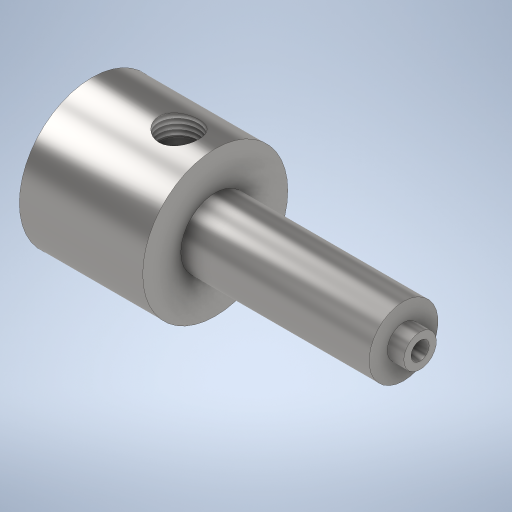
# Autodesk Inventor part: ASI Propane
Saved by Autodesk Inventor 2024 (Build 280153020, 153B)
## iProperties
Created: 2023-07-06
Part Number: ASI Propane
Material: Stainless Steel
Document SubType Name: Modeling
Designer: Victoria
Density: 8 g/cm^3
Appearance: Semi-Polished
Author: Victoria
Autodesk Inventor part; units mm, degrees
ref_plane "YZ Plane" through (0, 0, 0) normal (1, 0, 0) x (0, 1, 0)
ref_plane "XY Plane" through (0, 0, 0) normal (0, 0, 1) x (1, 0, 0)
sketch "Sketch1" plane through (0, 0, 0) normal (0, 0, 1) x (1, 0, 0)
  line L0 (0, 0) -> (0, 6.5)
  line L1 (0, 6.5) -> (54.81, 6.5)
  line L2 (67.887, 1.75) -> (54.81, 6.5)
  line L3 (71.47, 0) -> (71.47, 2.5)
  line L4 (71.47, 2.5) -> (67.887, 1.75)
  line L5 (0, 6.5) -> (0, 9.5)
  line L6 (0, 9.5) -> (60.7761, 9.5)
  line L7 (71.47, 0) -> (0, 0)
  line L8 (71.47, 2.5) -> (71.47, 4.5)
  line L9 (71.47, 4.5) -> (66.9088, 4.5)
  line L10 (66.9088, 4.5) -> (66.9088, 9.5)
  line L11 (66.9088, 9.5) -> (60.7761, 9.5)
  line L12 (66.9088, 9.5) -> (66.9088, 9.5)
  line L13 (66.9088, 9.5) -> (16.9088, 9.5)
  line L14 (16.9088, 9.5) -> (16.9088, 9.5)
  point P0 (71.47, 1.25)
  dimension "d0" = 6.5
  dimension "d1" = 54.81
  dimension "d5" = 2.5
  dimension "d6" = 3
  dimension "d7" = 0
  dimension "d8" = 50
  dimension "d44" = 1.75
  dimension "d45" = 3.583
  constraints: 30 end point, 7 perpendicular, 4 vertical, 1 horizontal, 1 midpoint, 1 point on line
  measures "d0" distance of L0.start L0.end
  measures "d1" distance of L0.end L1.end
  measures "d5" distance of L3.start L3.end
  measures "d6" distance of L0.end L5.end
  measures "d7" distance of L10.end L12.end
  measures "d8" distance of L12.end L13.end
  measures "d44" distance from line of L7 L2.start
  measures "d45" horizontal distance of point (71.47, 1.25) L2.start
revolve "Revolution1" add sketch "Sketch1" angle 360 about axis through (71.47, 0, 0) along (-1, 0, 0) contours L5 L6 L11 L10 L9 L8 L4 L2 L1
sketch "Sketch2" plane through (0, 0, 0) normal (-1, 0, 0) x (0, 0, 1)
  circle A0 centre (0, 0) radius 2.5 projected
  circle A1 centre (0, 0) radius 20
  circle A2 centre (0, 0) radius 6.5
  dimension "d10" = 40
  dimension "d11" = 13
  constraints: 2 centre point, 2 coincident
  measures "d10" diameter of A1
  measures "d11" diameter of A2
extrude "Extrusion1" add sketch "Sketch2" along normal blind 19 contours A1
sketch "Sketch3" plane through (0, 0, 0) normal (1, 0, 0) x (0, 0, -1)
  circle A0 centre (0, 0) radius 1.75 projected
  circle A1 centre (0, 0) radius 20
  circle A2 centre (0, 0) radius 4.5 projected
  circle A3 centre (0, 0) radius 9.5
  dimension "d18" = 40
  dimension "d37" = 19
  constraints: 2 centre point, 2 coincident
  measures "d18" diameter of A1
  measures "d37" diameter of A3
extrude "Extrusion2" add sketch "Sketch3" along normal blind 15 contours A1
sketch "Sketch4" plane through (0, 0, 0) normal (0, 1, 0) x (-1, 0, 0)
  line L0 (19, -20) -> (19, 20) projected
  line L1 (19, 0) -> (-5, 0)
  circle A0 centre (-5, 0) radius 1.75
  point P0 (0, 0)
  dimension "d21" = 24
  dimension "d22" = 3.5
  constraints: 2 end point, 1 centre point, 1 coincident, 1 horizontal, 1 midpoint
  measures "d21" distance of L1.start L1.end
  measures "d22" diameter of A0
extrude "Extrusion3" cut sketch "Sketch4" along normal through all both and the other way through all
ref_plane "Work Plane1" through (0, 20, 0) normal (0, 1, 0) x (-1, 0, 0)
sketch "Sketch5" plane through (0, 20, 0) normal (0, 1, 0) x (-1, 0, 0)
  line L0 (19, -20) -> (19, 20) projected
  line L1 (19, 0) -> (-5, 0)
  circle A0 centre (-5, 0) radius 3.175
  point P0 (0, 0)
  dimension "d26" = 24
  dimension "d27" = 6.35
  constraints: 2 end point, 1 centre point, 1 coincident, 1 horizontal, 1 midpoint
  measures "d26" distance of L1.start L1.end
  measures "d27" diameter of A0
hole "Hole1" at (5, 20, 0) direction (0, -1, 0) diameter 2 end through all counterbore diameter 11 counterbore depth 6
thread "Thread3" size "Rc 1/4" standard "BSP Taper Internal" length 11
mirror "Mirror1" about plane through (0, 0, 0) normal (0, 1, 0) of "Hole1"
thread "Thread4" size "M14x1.25" class "6H" standard "ANSI Metric M Profile" length 19
ref_plane "Work Plane3" through (0, 0, 0) normal (-1, 0, 0) x (0, 0, 1)
ref_plane "Work Plane2" through (0, 0, 0) normal (0, 1, 0) x (-1, 0, 0)
body "Solid1"
